yeet_spoiler (Autodesk Fusion 360 design; units mm, degrees)
Autodesk Fusion 360 part; units mm, degrees
note: some values were not read from the file. Set by a fixed rule: which sketch regions a step uses.
sketch "Sketch1" plane through (0, 0, 0) normal (0, 1, 0) x (1, 0, 0)
  line L0 (0, 0) -> (3.2805, -9.013)
  line L1 (4.69, -10) -> (5.6397, -10)
  line L2 (5.6397, -10) -> (2, 0)
  line L3 (2, 0) -> (0, 0)
  line L4 (3.2757, -9) -> (-16.7243, -9)
  line L5 (-16.7243, -9) -> (-20.921, 0)
  line L6 (-20.921, 0) -> (0, 0)
  line L7 (-15.0123, -1.9802) -> (-15.0129, -4.0929)
  line L8 (-15.0129, -4.0929) -> (-16.8525, -6.9995)
  line L9 (-16.8525, -6.9995) -> (-15.6643, -6.9998)
  line L10 (-15.6643, -6.9998) -> (-14.4824, -5.0142)
  line L11 (-14.4824, -5.0142) -> (-13.3256, -7.0005)
  line L12 (-13.3256, -7.0005) -> (-12.158, -7.0009)
  line L13 (-12.158, -7.0009) -> (-14.0028, -4.0864)
  line L14 (-14.0028, -4.0864) -> (-14.0021, -1.9805)
  line L15 (-14.0021, -1.9805) -> (-15.0123, -1.9802)
  line L16 (-11.6497, -1.9812) -> (-11.6512, -7.001)
  line L17 (-11.6512, -7.001) -> (-7.9292, -7.0021)
  line L18 (-7.9292, -7.0021) -> (-7.9289, -6.1529)
  line L19 (-7.9289, -6.1529) -> (-10.6374, -6.1521)
  line L20 (-10.6374, -6.1521) -> (-10.6371, -5.0393)
  line L21 (-10.6371, -5.0393) -> (-8.1169, -5.04)
  line L22 (-8.1169, -5.04) -> (-8.1167, -4.1943)
  line L23 (-8.1167, -4.1943) -> (-10.6368, -4.1935)
  line L24 (-10.6368, -4.1935) -> (-10.6364, -2.8273)
  line L25 (-10.6364, -2.8273) -> (-7.8321, -2.8281)
  line L26 (-7.8321, -2.8281) -> (-7.8318, -1.9823)
  line L27 (-7.8318, -1.9823) -> (-11.6497, -1.9812)
  line L28 (-6.9689, -1.9826) -> (-6.9704, -7.0024)
  line L29 (-6.9704, -7.0024) -> (-3.2484, -7.0035)
  line L30 (-3.2484, -7.0035) -> (-3.2481, -6.1543)
  line L31 (-3.2481, -6.1543) -> (-5.9566, -6.1535)
  line L32 (-5.9566, -6.1535) -> (-5.9563, -5.0407)
  line L33 (-5.9563, -5.0407) -> (-3.4361, -5.0414)
  line L34 (-3.4361, -5.0414) -> (-3.4359, -4.1956)
  line L35 (-3.4359, -4.1956) -> (-5.956, -4.1949)
  line L36 (-5.956, -4.1949) -> (-5.9556, -2.8287)
  line L37 (-5.9556, -2.8287) -> (-3.1512, -2.8295)
  line L38 (-3.1512, -2.8295) -> (-3.151, -1.9837)
  line L39 (-3.151, -1.9837) -> (-6.9689, -1.9826)
  line L40 (-1.1581, -1.9843) -> (-1.1594, -6.1549)
  line L41 (-1.1594, -6.1549) -> (-2.6489, -6.1545)
  line L42 (-2.6489, -6.1545) -> (-2.6491, -7.0037)
  line L43 (-2.6491, -7.0037) -> (1.34, -7.0049)
  line L44 (1.34, -7.0049) -> (1.3403, -6.1557)
  line L45 (1.3403, -6.1557) -> (-0.1458, -6.1552)
  line L46 (-0.1458, -6.1552) -> (-0.1446, -1.9846)
  line L47 (-0.1446, -1.9846) -> (-1.1581, -1.9843)
  arc A0 (3.2805, -9.013) -> (4.69, -10) centre (4.69, -8.5) ccw
  point P0 (3.6397, -10)
  dimension "d1" = 10
  dimension "d2" = 2
  dimension "d4" = 110
  dimension "d6" = 20
  dimension "d27" = 115
  dimension "d30" = 110
  dimension "d31" = 9
  dimension "d32" = 1.5
  constraint coincident L0.start L3.end
  constraint horizontal L1
  constraint parallel L0 L2
  constraint parallel L1 L3
  constraint coincident L0 L4.start
  constraint parallel L1 L4
  constraint coincident P0 L0
  constraint coincident P0 L1
  constraint tangent L0 A0
  constraint tangent L1 A0
  measures "d1" vertical distance of L1.end L2.end
  measures "d2" distance of P0 L1.end
  measures "d4" angle of L2 L6
  measures "d6" distance of L4.start L4.end
  measures "d27" angle of L5 L6
  measures "d30" angle of L0 L3
  measures "d31" distance of L4 L6
  measures "d32" radius of A0
extrude "Extrude1" add sketch "Sketch1" along normal blind 1.2 contours L0 L1 L2 L3 A0 | L0 L4 L5 L6 | L7 L8 L9 L10 L11 L12 L13 L14 L15 | L16 L17 L18 L19 L20 L21 L22 L23 L24 L25 L26 L27 | L28 L29 L30 L31 L32 L33 L34 L35 L36 L37 L38 L39 | L40 L41 L42 L43 L44 L45 L46 L47 makes body 1
extrude "Extrude2" add sketch "Sketch1" along normal blind 10 contours L0 L1 L2 L3 A0 bodies 1
ref_plane "WorkPlane1" through (0, 10, 0) normal (0, 1, 0) x (0, 0, 1)
mirror "Mirror1" about plane through (0, 10, 0) normal (0, 1, 0) of bodies 1 makes body 2
extrude "Extrude3" cut sketch "Sketch1" along normal blind 1.2 contours L7 L8 L9 L10 L11 L12 L13 L14 L15 | L16 L17 L18 L19 L20 L21 L22 L23 L24 L25 L26 L27 | L28 L29 L30 L31 L32 L33 L34 L35 L36 L37 L38 L39 | L40 L41 L42 L43 L44 L45 L46 L47 bodies 1
sketch "Sketch2" plane through (0, 20, 0) normal (0, 1, 0) x (-1, 0, 0)
  line L0 (16.7243, 9) -> (-3.2757, 9)
  line L1 (-3.2757, 9) -> (-3.2805, 9.013)
  line L2 (-4.69, 10) -> (-5.6397, 10)
  line L3 (-5.6397, 10) -> (-2, 0)
  line L4 (-2, 0) -> (20.921, 0)
  line L5 (20.921, 0) -> (16.7243, 9)
  line L6 (-0.1101, 2.02) -> (-0.1101, 4.18)
  line L7 (-0.1101, 4.18) -> (-1.99, 7.1522)
  line L8 (-1.99, 7.1522) -> (-0.7752, 7.1522)
  line L9 (-0.7752, 7.1522) -> (0.4326, 5.1217)
  line L10 (0.4326, 5.1217) -> (1.6158, 7.1522)
  line L11 (1.6158, 7.1522) -> (2.8096, 7.1522)
  line L12 (2.8096, 7.1522) -> (0.9227, 4.173)
  line L13 (0.9227, 4.173) -> (0.9227, 2.02)
  line L14 (0.9227, 2.02) -> (-0.1101, 2.02)
  line L15 (3.3277, 2.02) -> (3.3277, 7.1522)
  line L16 (3.3277, 7.1522) -> (7.1331, 7.1522)
  line L17 (7.1331, 7.1522) -> (7.1331, 6.284)
  line L18 (7.1331, 6.284) -> (4.364, 6.284)
  line L19 (4.364, 6.284) -> (4.364, 5.1462)
  line L20 (4.364, 5.1462) -> (6.9406, 5.1462)
  line L21 (6.9406, 5.1462) -> (6.9406, 4.2815)
  line L22 (6.9406, 4.2815) -> (4.364, 4.2815)
  line L23 (4.364, 4.2815) -> (4.364, 2.8847)
  line L24 (4.364, 2.8847) -> (7.2312, 2.8847)
  line L25 (7.2312, 2.8847) -> (7.2312, 2.02)
  line L26 (7.2312, 2.02) -> (3.3277, 2.02)
  line L27 (8.1134, 2.02) -> (8.1134, 7.1522)
  line L28 (8.1134, 7.1522) -> (11.9188, 7.1522)
  line L29 (11.9188, 7.1522) -> (11.9188, 6.284)
  line L30 (11.9188, 6.284) -> (9.1496, 6.284)
  line L31 (9.1496, 6.284) -> (9.1496, 5.1462)
  line L32 (9.1496, 5.1462) -> (11.7262, 5.1462)
  line L33 (11.7262, 5.1462) -> (11.7262, 4.2815)
  line L34 (11.7262, 4.2815) -> (9.1496, 4.2815)
  line L35 (9.1496, 4.2815) -> (9.1496, 2.8847)
  line L36 (9.1496, 2.8847) -> (12.0168, 2.8847)
  line L37 (12.0168, 2.8847) -> (12.0168, 2.02)
  line L38 (12.0168, 2.02) -> (8.1134, 2.02)
  line L39 (14.0543, 2.02) -> (14.0543, 6.284)
  line L40 (14.0543, 6.284) -> (12.5314, 6.284)
  line L41 (12.5314, 6.284) -> (12.5314, 7.1522)
  line L42 (12.5314, 7.1522) -> (16.6099, 7.1522)
  line L43 (16.6099, 7.1522) -> (16.6099, 6.284)
  line L44 (16.6099, 6.284) -> (15.0905, 6.284)
  line L45 (15.0905, 6.284) -> (15.0905, 2.02)
  line L46 (15.0905, 2.02) -> (14.0543, 2.02)
  arc A0 (-3.2805, 9.013) -> (-4.69, 10) centre (-4.69, 8.5) ccw
extrude "Extrude4" cut sketch "Sketch2" against normal blind 4 contours L6 L7 L8 L9 L10 L11 L12 L13 L14 | L15 L16 L17 L18 L19 L20 L21 L22 L23 L24 L25 L26 | L27 L28 L29 L30 L31 L32 L33 L34 L35 L36 L37 L38 | L39 L40 L41 L42 L43 L44 L45 L46 bodies 2
sketch "Sketch3" plane through (0, 10, 0) normal (0, 1, 0) x (1, 0, 0)
  line L0 (-15.5306, -11.5598) -> (-17.1245, -11.6992)
  line L1 (-17.1245, -11.6992) -> (-22.58, 0)
  line L2 (-22.58, 0) -> (-20.921, 0)
  line L3 (-20.921, 0) -> (-15.5306, -11.5598)
  line L4 (-20.921, 0) -> (0, 0)
  line L5 (-16.7243, -9) -> (-20.921, 0)
  dimension "d19" = 1.6
  dimension "d33" = 70
  constraint parallel L1 L3
  constraint coincident L2.end L3.start
  constraint collinear L2 L4
  constraint collinear L3 L5
  measures "d19" distance of L0.start L0.end
  measures "d33" angle of L0 L3
extrude "Extrude5" add sketch "Sketch3" along normal mid plane 50 bodies 1 2
fillet "Fillet1" radius 0.65 1 faces at (-16.5932, 18.3333, 11.6527) on bodies 1
sketch "Sketch4" plane through (0, 35, 0) normal (0, 1, 0) x (-1, 0, 0)
  line L0 (17.4169, 11.0723) -> (15.8645, 10.9365)
  arc A0 (15.8645, 10.9365) -> (15.9229, 10.7185) centre (16.512, 10.9932) ccw
  line L1 (15.9229, 10.7185) -> (20.921, 0)
  line L2 (20.921, 0) -> (22.58, 0)
  line L3 (22.58, 0) -> (17.4169, 11.0723)
  line L4 (19.8177, 0) -> (15.2145, 9.8714)
  line L5 (16.1523, 14.4163) -> (16.1928, 14.4352)
  line L6 (18.0638, 12.0512) -> (23.6834, 0)
  line L7 (23.6834, 0) -> (19.8177, 0)
  line L8 (20.921, 0) -> (0, 0)
  line L9 (16.7243, 9) -> (20.921, 0)
  spline S0 degree 5 poles (15.2145, 9.8714) (15.2028, 9.9133) (15.1798, 9.998) (15.1469, 10.1283) (15.1063, 10.3083) (15.0613, 10.544) (15.0228, 10.7901) (14.9925, 11.0459) (14.9732, 11.3105) (14.9689, 11.5821) (14.9842, 11.8579) (15.0238, 12.1337) (15.092, 12.4034) (15.1921, 12.6589) (15.3257, 12.8894) (15.4928, 13.0832) (15.6917, 13.2299) (15.9185, 13.3212) (16.1674, 13.3539) (16.4302, 13.3306) (16.6976, 13.2582) (16.96, 13.1458) (17.2086, 13.0033) (17.436, 12.8393) (17.6378, 12.6596) (17.8115, 12.4677) (17.9271, 12.3059) (18.0006, 12.1803) (18.0437, 12.0945) (18.0638, 12.0512) knots 0 0 0 0 0 0 0.04 0.08 0.12 0.16 0.2 0.24 0.28 0.32 0.36 0.4 0.44 0.48 0.52 0.56 0.6 0.64 0.68 0.72 0.76 0.8 0.84 0.88 0.92 0.96 1 1 1 1 1 1
  point P0 (15, 11)
  point P1 (15.1, 12.4)
  point P2 (15.9, 13.3)
  point P3 (17.2, 13)
  dimension "d28" = 1
  dimension "d29" = 1
  constraint perpendicular L4 L5
  constraint perpendicular L5 L6
  constraint parallel L3 L6
  constraint collinear L7 L8
  measures "d28" distance of L4 L9
  measures "d29" distance of L3 L6
extrude "Extrude6" add sketch "Sketch4" against normal blind 0.8 contours L0 A0 L1 L3 L4 L6 L7 L8 L9 S0 bodies 1
mirror "Mirror2" about plane through (0, 10, 0) normal (0, 1, 0) of "Extrude6"
sketch "Sketch6" plane through (-0.0006, 0, 1.9847) normal (-0.000295, 0, 1) x (0, -1, 0)
  line L0 (0, -11.6492) -> (0, -7.8312)
  line L1 (0, -7.8312) -> (-1.2, -7.8312)
  line L2 (-1.2, -7.8312) -> (-1.2, -11.6492)
  line L3 (-1.2, -11.6492) -> (0, -11.6492)
  line L4 (-1.2, -10.6492) -> (0, -10.6492)
  line L5 (0, -10.6492) -> (0, -10.2492)
  line L6 (0, -10.2492) -> (-1.2, -10.2492)
  line L7 (-1.2, -10.2492) -> (-1.2, -10.6492)
  dimension "d35" = 0.4
  dimension "d36" = 1
  constraint horizontal L4
  constraint vertical L5
  constraint horizontal L6
  constraint vertical L7
  constraint coincident L0 L5.end
  constraint coincident L2 L4.start
  measures "d35" distance of L4 L6
  measures "d36" distance of L3 L4
sketch "Sketch5" plane through (0, 0, 0) normal (-0.939793, 0, 0.341743) x (0, -1, 0)
  line L0 (0, 9.5766) -> (0, 10.6406)
  line L1 (0, 10.6406) -> (-20, 10.6406)
  line L2 (-20, 10.6406) -> (-20, 9.5766)
  line L3 (-20, 9.5766) -> (-18.8, 9.5766)
  line L4 (-18.8, 9.5766) -> (-18.8, 0)
  line L5 (-18.8, 0) -> (-1.2, 0)
  line L6 (-1.2, 0) -> (-1.2, 9.5766)
  line L7 (-1.2, 9.5766) -> (0, 9.5766)
